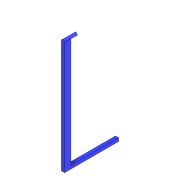
# Autodesk Inventor part: Bone15_14_Fix
Saved by Autodesk Inventor 2020 (Build 240168000, 168)
## iProperties
Created: 2021-03-17
Part Number: Bone15_14_Fix
Material: Generic
Document SubType Name: Modeling
Designer: deox
Density: 1 g/cm^3
Appearance: Blue - Wall Paint - Glossy
Author: deox
Autodesk Inventor part; units mm, degrees
ref_plane "YZ Plane" through (0, 0, 0) normal (1, 0, 0) x (0, 1, 0)
ref_plane "XZ Plane" through (0, 0, 0) normal (0, 1, 0) x (-1, 0, 0)
ref_plane "XY Plane" through (0, 0, 0) normal (0, 0, 1) x (1, 0, 0)
sketch "Sketch1" plane through (0, 0, 0) normal (0, 0, 1) x (1, 0, 0)
  circle A0 centre (0, 0) radius 0.05
  line L0 (0, 0) -> (0, -3.5)
  line L1 (-0.05, -3.55) -> (0.05, -3.55)
  line L2 (0.05, -3.55) -> (0.05, -3.45)
  line L3 (0.05, -3.45) -> (-0.05, -3.45)
  line L4 (-0.05, -3.45) -> (-0.05, -3.55)
  line L5 (-0.05, -3.55) -> (0.05, -3.45) construction
  line L6 (0.05, -3.55) -> (-0.05, -3.45) construction
  line L7 (0.05, -3.45) -> (0.05, 0)
  line L8 (-0.05, -3.45) -> (-0.05, 0)
  dimension "d0" = 0.1
  dimension "d1" = 3.5
  dimension "d2" = 0.1
  dimension "d3" = 0.1
  constraints: 18 end point, 2 midpoint, 2 parallel, 2 vertical, 1 coincident, 1 horizontal, 1 perpendicular, 1 symmetric about line, 3 other
  measures "d1" distance of L0.start L0.end
  measures "d2" distance of L3.end L2.end
  measures "d3" distance of L2.end L1.end
extrude "Extrusion1" add sketch "Sketch1" along normal blind 0.2
sketch "Sketch2" plane through (0, 0, 0) normal (0, 0, -1) x (-1, 0, 0)
  circle A0 centre (0, 0) radius 0.05
  dimension "d6" = 0.1
  constraints: 1 centre point, 1 coincident
  measures "d6" diameter of A0
extrude "Extrusion2" add sketch "Sketch2" along normal blind 0.2
sketch "Sketch3" plane through (0, 0, 0) normal (0, 0, -1) x (-1, 0, 0)
  line L0 (0.05, -3.55) -> (-0.05, -3.55) projected
  line L1 (-0.05, -3.55) -> (0.05, -3.55)
  line L2 (0.05, -3.55) -> (0.05, -3.45)
  line L3 (0.05, 0) -> (0.05, -3.55) projected
  line L4 (0.05, -3.45) -> (-0.05, -3.45)
  line L5 (-0.05, -3.55) -> (-0.05, 0) projected
  line L6 (-0.05, -3.45) -> (-0.05, -3.55)
  point P0 (0, 0)
  dimension "d9" = 0.1
  constraints: 8 end point, 2 perpendicular, 2 point on line, 1 collinear
  measures "d9" distance of L0.start L2.end
extrude "Extrusion3" add sketch "Sketch3" along normal blind 1.5
body "Solid1"
